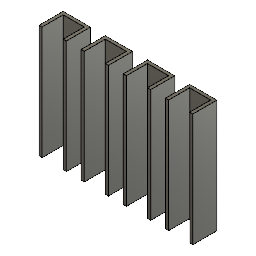
Cable_covers (Autodesk Fusion 360 design; units mm, degrees)
Autodesk Fusion 360 part; units mm, degrees
sketch "Sketch1" plane through (0, 0, 0) normal (0, 1, 0) x (1, 0, 0)
  line L0 (0, 0) -> (0, 23)
  line L1 (0, 23) -> (26, 23)
  line L2 (0, 0) -> (3, 0)
  line L3 (23, 20) -> (3, 20)
  line L4 (3, 20) -> (3, 0)
  line L5 (23, 20) -> (23, 0)
  line L6 (26, 23) -> (26, 0)
  line L7 (26, 0) -> (23, 0)
  dimension "d1" = 23
  dimension "d2" = 26
  dimension "d3" = 3
  constraint coincident L0.start L2.start
  constraint vertical L0
  constraint perpendicular L0 L1
  constraint horizontal L2
  constraint perpendicular L2 L4
  constraint perpendicular L3 L5
  constraint perpendicular L1 L6
  constraint perpendicular L5 L7
  measures "d1" distance of L0.start L0.end
  measures "d2" distance of L0.end L1.end
  measures "d3" distance of L0.start L2.end
extrude "Extrude1" add sketch "Sketch1" along normal blind 107.5 makes body 1
pattern_linear "R-Pattern1" count 4 spacing 40 along (1, 0, 0) both ways of bodies 1 makes body 2 at (-31.3333, 35.8333, -23) makes body 3 at (48.6667, 35.8333, -23) makes body 4 at (88.6667, 35.8333, -23)
equation "d4 = ( 21.5 / 2 ) * 1 cm"
